Autodesk Inventor part; units mm, degrees
(part 2 of 2)
sketch "Skizze3" plane through (0, 0, 0) normal (0, 0, -1) x (-1, 0, 0)
  circle A0 centre (-92.4124, -26) radius 3 projected
  circle A1 centre (-92.4124, -46) radius 3 projected
  circle A2 centre (-82.4124, -46) radius 3 projected
  circle A3 centre (-82.4124, -26) radius 3 projected
  circle A4 centre (-74.4124, -26) radius 3 projected
  circle A5 centre (-74.4124, -46) radius 3 projected
  circle A6 centre (-64.4124, -46) radius 3 projected
  circle A7 centre (-64.4124, -26) radius 3 projected
  circle A8 centre (-56.4124, -26) radius 3 projected
  circle A9 centre (-56.4124, -46) radius 3 projected
  circle A10 centre (-46.4124, -46) radius 3 projected
  circle A11 centre (-46.4124, -26) radius 3 projected
  circle A12 centre (-38.4124, -26) radius 3 projected
  circle A13 centre (-38.4124, -46) radius 3 projected
  circle A14 centre (-28.4124, -46) radius 3 projected
  circle A15 centre (-28.4124, -26) radius 3 projected
  circle A16 centre (-20.4124, -26) radius 3 projected
  circle A17 centre (-20.4124, -46) radius 3 projected
  circle A18 centre (-10.4124, -46) radius 3 projected
  circle A19 centre (-10.4124, -26) radius 3 projected
  circle A20 centre (-2.4124, -26) radius 3 projected
  circle A21 centre (-2.4124, -46) radius 3 projected
  circle A22 centre (7.5876, -46) radius 3 projected
  circle A23 centre (7.5876, -26) radius 3 projected
  circle A24 centre (-92.4124, 10) radius 3 projected
  circle A25 centre (-92.4124, -10) radius 3 projected
  circle A26 centre (-82.4124, -10) radius 3 projected
  circle A27 centre (-82.4124, 10) radius 3 projected
  circle A28 centre (-74.4124, 10) radius 3 projected
  circle A29 centre (-74.4124, -10) radius 3 projected
  circle A30 centre (-64.4124, -10) radius 3 projected
  circle A31 centre (-64.4124, 10) radius 3 projected
  circle A32 centre (-56.4124, 10) radius 3 projected
  circle A33 centre (-56.4124, -10) radius 3 projected
  circle A34 centre (-46.4124, -10) radius 3 projected
  circle A35 centre (-46.4124, 10) radius 3 projected
  circle A36 centre (-38.4124, 10) radius 3 projected
  circle A37 centre (-38.4124, -10) radius 3 projected
  circle A38 centre (-28.4124, -10) radius 3 projected
  circle A39 centre (-28.4124, 10) radius 3 projected
  circle A40 centre (-20.4124, 10) radius 3 projected
  circle A41 centre (-20.4124, -10) radius 3 projected
  circle A42 centre (-10.4124, -10) radius 3 projected
  circle A43 centre (-10.4124, 10) radius 3 projected
  circle A44 centre (-2.4124, 10) radius 3 projected
  circle A45 centre (-2.4124, -10) radius 3 projected
  circle A46 centre (7.5876, -10) radius 3 projected
  circle A47 centre (7.5876, 10) radius 3 projected
  line L0 (15.5959, 21.9352) -> (-100.3476, 21.9352) projected
  line L1 (-100.3476, 21.9352) -> (-100.3476, -57.9) projected
  line L2 (-100.3476, -57.9) -> (15.5959, -57.9) projected
  line L3 (15.5959, -57.9) -> (15.5959, 21.9352) projected
  line L4 (-96.8476, -54.4) -> (-96.8476, 18.4352)
  line L5 (-96.8476, 18.4352) -> (12.0959, 18.4352)
  line L6 (12.0959, 18.4352) -> (12.0959, -54.4)
  line L7 (12.0959, -54.4) -> (-96.8476, -54.4)
  point P0 (0, 0)
  dimension "d16" = 3.5
  constraints: 8 end point, 3 other
  measures "d16" distance between parallel lines of L1 L4
ref_plane "Arbeitsebene2" through (47.4124, 4.95, -60.9) normal (0, 0, -1) x (0, 1, 0)
ref_plane "Arbeitsebene3" through (61.7974, -12.65, -54) normal (0, 0, -1) x (0, 1, 0)
ref_plane "Arbeitsebene4" through (78.5124, -53.9, -59.1) normal (0, 0, -1) x (0, 1, 0)
extrude "Extrusion2" add sketch "Skizze3" along normal up to surface (59.1 mm away) contours L3 L2 L1 L0
sketch "Skizze4" plane through (-15.5959, -57.9, 4) normal (0, -1, 0) x (1, 0, 0)
  line L0 (115.9434, 0) -> (115.9434, -63.1) projected
  line L1 (0, 0) -> (115.9434, 0) projected
  line L2 (0, 0) -> (0, -63.1) projected
  line L3 (0, -63.1) -> (115.9434, -63.1) projected
  line L4 (105.9434, -49.1) -> (105.9434, -14)
  line L5 (101.9434, -10) -> (14, -10)
  line L6 (10, -14) -> (10, -49.1)
  line L7 (14, -53.1) -> (101.9434, -53.1)
  arc A0 (101.9434, -53.1) -> (105.9434, -49.1) centre (101.9434, -49.1) ccw
  arc A1 (10, -49.1) -> (14, -53.1) centre (14, -49.1) ccw
  arc A2 (14, -10) -> (10, -14) centre (14, -14) ccw
  arc A3 (105.9434, -14) -> (101.9434, -10) centre (101.9434, -14) ccw
  point P0 (15.5959, -4)
  point P1 (105.9434, -53.1)
  point P2 (105.9434, -10)
  point P3 (10, -10)
  point P4 (10, -53.1)
  dimension "d19" = 10
  dimension "d22" = 4
  constraints: 8 end point, 8 point on circle, 8 point on line, 8 tangent, 4 centre point, 3 equal radius, 3 other
  measures "d19" distance between parallel lines of L3 L7
  measures "d22" radius of A0
extrude "Extrusion3" cut sketch "Skizze4" against normal through all contours A0 L7 A1 L6 A2 L5 A3 L4
sketch "Skizze5" plane through (-15.5959, -57.9, 4) normal (-1, 0, 0) x (0, 0, 1)
  line L0 (0, 0) -> (-63.1, 0) projected
  line L1 (0, 79.8352) -> (0, 0) projected
  line L2 (-63.1, 79.8352) -> (0, 79.8352) projected
  line L3 (-63.1, 79.8352) -> (-63.1, 0) projected
  line L4 (-51.1, 8) -> (-12, 8)
  line L5 (-8, 12) -> (-8, 67.8352)
  line L6 (-12, 71.8352) -> (-51.1, 71.8352)
  line L7 (-55.1, 67.8352) -> (-55.1, 12)
  arc A0 (-55.1, 12) -> (-51.1, 8) centre (-51.1, 12) ccw
  arc A1 (-51.1, 71.8352) -> (-55.1, 67.8352) centre (-51.1, 67.8352) ccw
  arc A2 (-8, 67.8352) -> (-12, 71.8352) centre (-12, 67.8352) ccw
  arc A3 (-12, 8) -> (-8, 12) centre (-12, 12) ccw
  point P0 (-4, 57.9)
  dimension "d23" = 8
  dimension "d24" = 4
  constraints: 8 end point, 8 point on circle, 8 tangent, 4 centre point, 3 equal radius, 3 other
  measures "d23" distance between parallel lines of L0 L4
  measures "d24" radius of A0
extrude "Extrusion4" cut sketch "Skizze5" against normal through all contours A0 L7 A1 L6 A2 L5 A3 L4
fillet "Rundung1" radius 4 4 edges at (-15.5959, -57.9, -27.55) (-15.5959, 21.9352, -27.55) (100.3476, 21.9352, -27.55) (100.3476, -57.9, -27.55)
sketch "Skizze6" plane through (96.3476, -57.9, -59.1) normal (0, 0, -1) x (-1, 0, 0)
  line L0 (108.4434, 76.3352) -> (-0.5, 76.3352) projected
  line L1 (108.4434, 3.5) -> (108.4434, 76.3352) projected
  line L2 (-0.5, 3.5) -> (108.4434, 3.5) projected
  line L3 (-0.5, 76.3352) -> (-0.5, 3.5) projected
  arc A0 (-4, 4) -> (0, 0) centre (0, 4) ccw projected
  line L4 (107.9434, 0) -> (0, 0) projected
  arc A1 (107.9434, 0) -> (111.9434, 4) centre (107.9434, 4) ccw projected
  line L5 (111.9434, 75.8352) -> (111.9434, 4) projected
  arc A2 (111.9434, 75.8352) -> (107.9434, 79.8352) centre (107.9434, 75.8352) ccw projected
  line L6 (0, 79.8352) -> (107.9434, 79.8352) projected
  arc A3 (0, 79.8352) -> (-4, 75.8352) centre (0, 75.8352) ccw projected
  line L7 (-4, 4) -> (-4, 75.8352) projected
  line L8 (109.9717, 6.4176) -> (-2.0283, 6.4176) construction
  line L9 (-2.0283, 6.4176) -> (-2.0283, 73.4176) construction
  line L10 (-2.0283, 73.4176) -> (109.9717, 73.4176) construction
  line L11 (109.9717, 73.4176) -> (109.9717, 6.4176) construction
  line L12 (109.9717, 6.4176) -> (-2.0283, 73.4176) construction
  line L13 (-2.0283, 6.4176) -> (109.9717, 73.4176) construction
  line L14 (106.4717, 1.9176) -> (1.4717, 1.9176) construction
  line L15 (1.4717, 1.9176) -> (1.4717, 77.9176) construction
  line L16 (1.4717, 77.9176) -> (106.4717, 77.9176) construction
  line L17 (106.4717, 77.9176) -> (106.4717, 1.9176) construction
  line L18 (106.4717, 1.9176) -> (1.4717, 77.9176) construction
  line L19 (1.4717, 1.9176) -> (106.4717, 77.9176) construction
  point P0 (96.3476, 57.9)
  point P1 (53.9717, 39.9176)
  point P2 (53.9717, 39.9176)
  dimension "d28" = 112
  dimension "d29" = 67
  dimension "d30" = 105
  dimension "d31" = 76
  constraints: 24 end point, 5 midpoint, 4 parallel, 2 horizontal, 2 perpendicular
  measures "d28" distance of L9.end L10.end
  measures "d29" distance of L8.end L9.end
  measures "d30" distance of L15.end L16.end
  measures "d31" distance of L14.end L15.end
hole "Bohrung2" at (-10.1241, 20.0176, -59.1) at (-13.6241, 15.5176, -59.1) at (-13.6241, -51.4824, -59.1) at (-10.1241, -55.9824, -59.1) at (94.8759, -55.9824, -59.1) at (98.3759, -51.4824, -59.1) at (98.3759, 15.5176, -59.1) at (94.8759, 20.0176, -59.1) direction (0, 0, 1) diameter 1.8 depth 12 tip angle 118
sketch "Skizze7" plane through (0, 0, 4) normal (0, 0, 1) x (1, 0, 0)
  circle A0 centre (87.4124, -27.05) radius 3.95 projected
  circle A1 centre (87.4124, -44.95) radius 3.95 projected
  circle A2 centre (87.4124, 8.95) radius 3.95 projected
  circle A3 centre (87.4124, -8.95) radius 3.95 projected
  circle A4 centre (69.4124, -27.05) radius 3.95 projected
  circle A5 centre (69.4124, -44.95) radius 3.95 projected
  circle A6 centre (69.4124, 8.95) radius 3.95 projected
  circle A7 centre (69.4124, -8.95) radius 3.95 projected
  circle A8 centre (51.4124, -27.05) radius 3.95 projected
  circle A9 centre (51.4124, -44.95) radius 3.95 projected
  circle A10 centre (51.4124, 8.95) radius 3.95 projected
  circle A11 centre (51.4124, -8.95) radius 3.95 projected
  circle A12 centre (33.4124, -27.05) radius 3.95 projected
  circle A13 centre (33.4124, -44.95) radius 3.95 projected
  circle A14 centre (33.4124, 8.95) radius 3.95 projected
  circle A15 centre (33.4124, -8.95) radius 3.95 projected
  circle A16 centre (15.4124, -27.05) radius 3.95 projected
  circle A17 centre (15.4124, -44.95) radius 3.95 projected
  circle A18 centre (15.4124, 8.95) radius 3.95 projected
  circle A19 centre (15.4124, -8.95) radius 3.95 projected
  circle A20 centre (-2.5876, -27.05) radius 3.95 projected
  circle A21 centre (-2.5876, -44.95) radius 3.95 projected
  circle A22 centre (15.4124, 0) radius 3 projected
  circle A23 centre (51.4124, 0) radius 3 projected
  circle A24 centre (87.4124, 0) radius 3 projected
  circle A25 centre (69.4124, -36) radius 3 projected
  circle A26 centre (33.4124, -36) radius 3 projected
  circle A27 centre (-2.5876, -36) radius 3 projected
  circle A28 centre (15.4124, -36) radius 3 projected
  circle A29 centre (51.4124, -36) radius 3 projected
  circle A30 centre (87.4124, -36) radius 3 projected
  circle A31 centre (69.4124, 0) radius 3 projected
  circle A32 centre (33.4124, 0) radius 3 projected
  circle A33 centre (-2.5876, 0) radius 3 projected
  circle A34 centre (-2.5876, 8.95) radius 3.95 projected
  circle A35 centre (-2.5876, -8.95) radius 3.95 projected
  circle A36 centre (98.3759, 15.5176) radius 0.9 projected
  circle A37 centre (94.8759, -55.9824) radius 0.9 projected
  circle A38 centre (-13.6241, -51.4824) radius 0.9 projected
  circle A39 centre (-10.1241, 20.0176) radius 0.9 projected
  circle A40 centre (-13.6241, 15.5176) radius 0.9 projected
  circle A41 centre (-10.1241, -55.9824) radius 0.9 projected
  circle A42 centre (98.3759, -51.4824) radius 0.9 projected
  circle A43 centre (94.8759, 20.0176) radius 0.9 projected
  arc A44 (96.3476, -57.9) -> (100.3476, -53.9) centre (96.3476, -53.9) ccw projected
  line L0 (96.3476, -57.9) -> (-11.5959, -57.9) projected
  arc A45 (-15.5959, -53.9) -> (-11.5959, -57.9) centre (-11.5959, -53.9) ccw projected
  line L1 (-15.5959, -53.9) -> (-15.5959, 17.9352) projected
  arc A46 (-11.5959, 21.9352) -> (-15.5959, 17.9352) centre (-11.5959, 17.9352) ccw projected
  line L2 (-11.5959, 21.9352) -> (96.3476, 21.9352) projected
  arc A47 (100.3476, 17.9352) -> (96.3476, 21.9352) centre (96.3476, 17.9352) ccw projected
  line L3 (100.3476, 17.9352) -> (100.3476, -53.9) projected
  point P0 (0, 0)
extrude "Extrusion5" cut sketch "Skizze7" against normal blind 10 contours A36 | A37 | A38 | A39 | A40 | A41 | A42 | A43
sketch "Skizze8" plane through (-11.5959, -57.9, 4) normal (0, -1, 0) x (1, 0, 0)
  circle A0 centre (104.4434, -19.0756) radius 0.9 projected
  circle A1 centre (104.4434, -40.1278) radius 0.9 projected
  line L0 (101.9434, -47.0289) -> (101.9434, -14) projected
  line L1 (101.9434, -47.0289) -> (106.9434, -47.0289) projected
  line L2 (106.9434, -14) -> (106.9434, -47.0289) projected
  line L3 (101.9434, -14) -> (106.9434, -14) projected
  line L4 (107.9434, 0) -> (107.9434, -63.1) projected
  line L5 (0, 0) -> (107.9434, 0) projected
  line L6 (0, -63.1) -> (0, 0) projected
  line L7 (0, -63.1) -> (107.9434, -63.1) projected
  arc A2 (97.9434, -53.1) -> (101.9434, -49.1) centre (97.9434, -49.1) ccw projected
  line L8 (97.9434, -53.1) -> (10, -53.1) projected
  arc A3 (6, -49.1) -> (10, -53.1) centre (10, -49.1) ccw projected
  line L9 (6, -49.1) -> (6, -14) projected
  arc A4 (10, -10) -> (6, -14) centre (10, -14) ccw projected
  line L10 (10, -10) -> (97.9434, -10) projected
  arc A5 (101.9434, -14) -> (97.9434, -10) centre (97.9434, -14) ccw projected
  line L11 (101.9434, -14) -> (101.9434, -49.1) projected
  circle A6 centre (3.5, -40.1278) radius 0.9
  circle A7 centre (3.5, -14) radius 0.9
  point P0 (11.5959, -4)
  dimension "d41" = 1.8
  dimension "d42" = 1.8
  dimension "d43" = 2.5
  dimension "d44" = 2.5
  constraints: 2 centre point
  measures "d41" diameter of A6
  measures "d42" diameter of A7
  measures "d43" distance from line of A6.centre L9
  measures "d44" distance from line of L9 A7.centre
extrude "Extrusion6" cut sketch "Skizze8" against normal blind 10 contours A0 | A1 | A6 | A7
